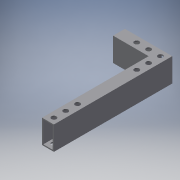
# Autodesk Inventor part: right arm
Saved by Autodesk Inventor 2018 (Build 220112000, 112)
## iProperties
Created: 2019-01-16
Part Number: right arm
Material: Generic
Document SubType Name: Modeling
Designer: s-4008082
Density: 1 g/cm^3
Appearance: Default
Author: s-4008082
Autodesk Inventor part; units mm, degrees
ref_plane "YZ Plane" through (0, 0, 0) normal (1, 0, 0) x (0, 1, 0)
ref_plane "XZ Plane" through (0, 0, 0) normal (0, 1, 0) x (-1, 0, 0)
ref_plane "XY Plane" through (0, 0, 0) normal (0, 0, 1) x (1, 0, 0)
sketch "Sketch15" plane through (0, 0, 0) normal (1, 0, 0) x (0, 1, 0)
  line L0 (0, 0) -> (50.8, 0)
  line L1 (50.8, 0) -> (50.8, 25.4)
  line L2 (50.8, 25.4) -> (0, 25.4)
  line L3 (0, 25.4) -> (0, 0)
  line L4 (48.26, 22.86) -> (2.54, 22.86)
  line L5 (2.54, 22.86) -> (2.54, 2.54)
  line L6 (2.54, 2.54) -> (48.26, 2.54)
  line L7 (48.26, 2.54) -> (48.26, 22.86)
  dimension "d46" = 25.4
  dimension "d47" = 50.8
  dimension "d48" = 2.54
  dimension "d49" = 2.54
  dimension "d50" = 2.54
  dimension "d51" = 2.54
  constraints: 16 end point, 4 parallel, 2 horizontal, 2 perpendicular
  measures "d46" distance of L0.end L1.end
  measures "d47" distance of L1.end L2.end
  measures "d48" distance between parallel lines of L1 L7
  measures "d49" distance between parallel lines of L2 L4
  measures "d50" distance between parallel lines of L3 L5
  measures "d51" distance between parallel lines of L0 L6
extrude "Extrusion12" add sketch "Sketch15" along normal blind 76.2
sketch "Sketch16" plane through (0, 0, 0) normal (0, 0, -1) x (-1, 0, 0)
  line L0 (0, 0) -> (-76.2, 0) projected
  line L1 (-76.2, 0) -> (-101.6, 0)
  line L2 (-101.6, 0) -> (-101.6, 50.8)
  line L3 (-101.6, 50.8) -> (-76.2, 50.8)
  line L4 (-76.2, 50.8) -> (-76.2, 0)
  line L5 (-78.74, 48.26) -> (-99.06, 48.26)
  line L6 (-99.06, 48.26) -> (-99.06, 2.54)
  line L7 (-99.06, 2.54) -> (-78.74, 2.54)
  line L8 (-78.74, 2.54) -> (-78.74, 48.26)
  dimension "d54" = 25.4
  dimension "d55" = 50.8
  dimension "d56" = 2.54
  dimension "d57" = 2.54
  dimension "d58" = 2.54
  dimension "d59" = 2.54
  constraints: 16 end point, 4 parallel, 2 horizontal, 2 perpendicular
  measures "d54" distance of L2.end L3.end
  measures "d55" distance of L1.end L2.end
  measures "d56" distance between parallel lines of L3 L5
  measures "d57" distance between parallel lines of L2 L6
  measures "d58" distance between parallel lines of L1 L7
  measures "d59" distance between parallel lines of L4 L8
extrude "Extrusion13" add sketch "Sketch16" against normal blind 254
sketch "Sketch17" plane through (0, 0, 0) normal (0, 0, -1) x (-1, 0, 0)
  line L0 (0, 2.54) -> (-76.2, 2.54) projected
  line L1 (0, 48.26) -> (-76.2, 48.26) projected
  line L2 (-73.617, 2.54) -> (-3.1161, 2.54)
  line L3 (-3.1161, 2.54) -> (-3.1161, 48.26)
  line L4 (-3.1161, 48.26) -> (-73.617, 48.26)
  line L5 (-73.617, 48.26) -> (-73.617, 2.54)
  point P0 (0, 0)
  constraints: 8 end point, 2 parallel, 2 point on line, 1 horizontal, 1 perpendicular
extrude "Extrusion14" add sketch "Sketch17" along normal blind 2.54
sketch "Sketch20" plane through (0, 0, 0) normal (0, -1, 0) x (1, 0, 0)
  circle A0 centre (88.9, 12.7) radius 5.2917
  circle A1 centre (63.5, 12.7) radius 5.2917
  circle A2 centre (38.1, 12.7) radius 5.2917
  line L0 (0, 25.4) -> (76.2, 25.4) projected
  circle A3 centre (88.9, 38.1) radius 5.2917
  circle A4 centre (88.9, 63.5) radius 5.2917
  line L1 (76.2, 25.4) -> (76.2, 254) projected
  line L2 (101.6, 0) -> (101.6, 254) projected
  point P0 (0, 0)
  dimension "d71" = 12.7
  dimension "d72" = 12.7
  dimension "d73" = 12.7
  dimension "d74" = 10.5833
  dimension "d75" = 10.5833
  dimension "d76" = 10.5833
  dimension "d77" = 12.7
  dimension "d78" = 12.7
  dimension "d79" = 10.5833
  dimension "d80" = 10.5833
  dimension "d81" = 12.7
  dimension "d82" = 25.4
  dimension "d83" = 25.4
  dimension "d84" = 25.4
  dimension "d85" = 25.4
  constraints: 5 centre point
  measures "d71" distance from line of L0 A2.centre
  measures "d72" distance from line of L0 A1.centre
  measures "d73" distance from line of L0 A0.centre
  measures "d74" diameter of A2
  measures "d75" diameter of A1
  measures "d76" diameter of A0
  measures "d77" distance from line of L1 A3.centre
  measures "d78" distance from line of L1 A4.centre
  measures "d79" diameter of A4
  measures "d80" diameter of A3
  measures "d81" distance from line of L2 A0.centre
  measures "d82" distance of A3.centre A0.centre
  measures "d83" distance of A3.centre A4.centre
  measures "d84" distance of A0.centre A1.centre
  measures "d85" distance of A1.centre A2.centre
extrude "Extrusion16" cut sketch "Sketch20" against normal blind 76.2
sketch "Sketch21" plane through (0, 50.8, 25.4) normal (0, 1, 0) x (1, 0, 0)
  circle A0 centre (88.9, -215.9) radius 5.2917
  circle A1 centre (88.9, -190.5) radius 5.2917
  circle A2 centre (88.9, -165.1) radius 5.2917
  line L0 (101.6, -228.6) -> (76.2, -228.6) projected
  line L1 (76.2, 0) -> (76.2, -228.6) projected
  point P0 (0, 25.4)
  dimension "d88" = 10.5833
  dimension "d89" = 10.5833
  dimension "d90" = 10.5833
  dimension "d91" = 25.4
  dimension "d92" = 25.4
  dimension "d93" = 12.7
  dimension "d94" = 12.7
  dimension "d95" = 12.7
  dimension "d96" = 12.7
  constraints: 3 centre point
  measures "d88" diameter of A0
  measures "d89" diameter of A1
  measures "d90" diameter of A2
  measures "d91" distance of A1.centre A2.centre
  measures "d92" distance of A0.centre A1.centre
  measures "d93" distance from line of L0 A0.centre
  measures "d94" distance from line of L1 A0.centre
  measures "d95" distance from line of L1 A1.centre
  measures "d96" distance from line of L1 A2.centre
extrude "Extrusion17" cut sketch "Sketch21" against normal blind 76.2
equation "\"d49\" = d48"
equation "\"d50\" = d48"
equation "\"d51\" = d48"
equation "\"d56\" = d48"
equation "\"d57\" = d48"
equation "\"d58\" = d48"
equation "\"d59\" = d48"
equation "\"d72\" = d71"
equation "\"d73\" = d71"
equation "\"d75\" = d74"
equation "\"d76\" = d74"
equation "\"d77\" = d71"
equation "\"d78\" = d71"
equation "\"d79\" = d74"
equation "\"d80\" = d74"
equation "\"d81\" = d71"
equation "\"d83\" = d82"
equation "\"d84\" = d82"
equation "\"d85\" = d82"
equation "\"d92\" = d91"
body "Solid2"
